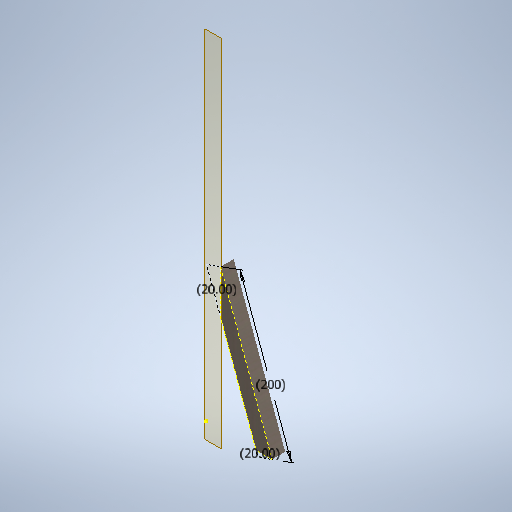
# Autodesk Inventor part: BaseAngularSmall
Saved by Autodesk Inventor 2025.2 (Build 292293000, 293)
## iProperties
Created: 2025-03-06
Part Number: BaseAngularSmall
Material: Wood (Walnut)
Document SubType Name: Modeling
Designer: baolo
Density: 0.55 g/cm^3
Appearance: Walnut
Author: baolo
Autodesk Inventor part; units mm, degrees
ref_plane "YZ Plane" through (0, 0, 0) normal (1, 0, 0) x (0, 1, 0)
ref_plane "XZ Plane" through (0, 0, 0) normal (0, 1, 0) x (-1, 0, 0)
ref_plane "XY Plane" through (0, 0, 0) normal (0, 0, 1) x (1, 0, 0)
ref_plane "Work Plane1" through (0, 0, 0) normal (0, 0, 1) x (1, 0, 0)
sketch "Sketch1" plane through (0, 0, 0) normal (0, 0, 1) x (1, 0, 0)
  line L0 (20, 0) -> (20, 430) construction
  line L1 (20, 0) -> (100, 0) construction
  line L2 (67.1205, 0) -> (88.404, 0)
  line L3 (88.404, 0) -> (20, 187.9385)
  line L4 (20, 187.9385) -> (20, 129.4624)
  line L5 (20, 129.4624) -> (67.1205, 0)
  line L6 (43.5602, 64.7312) -> (62.3541, 71.5716) construction
  line L7 (100, 0) -> (100, -20) construction
  line L8 (1.2061, 181.0981) -> (20, 129.4624) construction
  line L9 (67.1205, 0) -> (69.6102, -6.8404) construction
  line L10 (69.6102, -6.8404) -> (88.404, 0) construction
  line L11 (20, 187.9385) -> (1.2061, 181.0981) construction
  point P0 (0, 0)
  dimension "d0" = 70
  dimension "d5" = 200
  constraints: 18 end point, 5 perpendicular, 5 point on line, 2 equal length, 1 midpoint
  measures "d0" angle of L1 L5
  measures "d5" distance of L2.end L3.end
ref_plane "Work Plane2" through (0, 0, -20) normal (0, 0, -1) x (0, 1, 0)
ref_plane "Work Plane3" through (20, -17.4625, -17.4625) normal (0, 0, -1) x (0, 1, 0)
extrude "Extrusion1" add sketch "Sketch1" against normal up to surface (17.4625 mm away)
sketch "Sketch2" plane through (0, 0, 0) normal (0, 0, 1) x (1, 0, 0)
  line L0 (88.404, 0) -> (20, 187.9385) construction
  line L1 (20, 187.9385) -> (20, 129.4624) construction
  line L2 (20, 129.4624) -> (67.1205, 0) construction
  line L3 (67.1205, 0) -> (88.404, 0) construction
  line L4 (20, 187.9385) -> (1.2061, 181.0981) construction
  line L5 (1.2061, 181.0981) -> (20, 129.4624) construction
  line L6 (88.404, 0) -> (69.6102, -6.8404) construction
  line L7 (69.6102, -6.8404) -> (67.1205, 0) construction
  line L8 (20, 129.4624) -> (67.1205, 0) construction
  point P0 (0, 0)
  dimension "d6" = 200
  dimension "d7" = 20
  dimension "d8" = 20
  constraints: 8 end point, 2 collinear, 2 perpendicular
  measures "d6" distance between parallel lines of L6 L4
  measures "d7" angle of L5 L1
  measures "d8" angle of L6 L3
body "Solid1"
